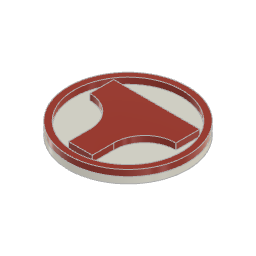
_T.1f97fbe8-ec46-4ea8-aa97-27b6090c93b7 (Autodesk Fusion 360 design; units mm, degrees)
Autodesk Fusion 360 part; units mm, degrees
sketch "Sketch1" plane through (0, 0, 0) normal (0, 0, 1) x (1, 0, 0)
  circle A0 centre (0, 0) radius 15.875
  circle A1 centre (0, 0) radius 14.2875
  line L0 (3.175, -12.7) -> (0, -12.7)
  line L1 (0, -12.7) -> (-3.175, -12.7)
  line L2 (-3.175, -12.7) -> (3.175, -12.7)
  line L3 (3.175, -12.7) -> (3.175, 3.6501)
  line L4 (3.175, 3.6501) -> (-3.175, 3.6501)
  line L5 (-3.175, 3.6501) -> (-3.175, -12.7)
  line L6 (-11.43, 7.62) -> (11.4939, 7.62)
  line L7 (11.4939, 7.62) -> (11.4939, 1.27)
  line L8 (11.4939, 1.27) -> (-11.43, 1.27)
  line L9 (-11.43, 1.27) -> (-11.43, 7.62)
  line L10 (-11.43, 1.27) -> (0.2443, 1.27) construction
  arc A2 (-3.175, -6.985) -> (-11.43, 1.27) centre (-11.43, -6.985) ccw
  line L11 (0, -12.7) -> (0, -11.684)
  arc A3 (11.43, 1.27) -> (3.175, -6.985) centre (11.43, -6.985) ccw
  dimension "d5" = 3.175
  dimension "d16" = 6.35
  constraint coincident A0.centre A1.centre
  constraint horizontal L0
  constraint horizontal L1
  constraint horizontal L2
  constraint vertical L3
  constraint horizontal L4
  constraint vertical L5
  constraint horizontal L6
  constraint vertical L7
  constraint horizontal L8
  constraint vertical L9
  constraint horizontal L10
  constraint coincident L5 A2.start
  constraint tangent L5 A2
  constraint tangent L8 A2
  constraint perpendicular L1 L11
  constraint symmetric L8.end L11 A3.start
  constraint symmetric A2.start L11 A3.end
  constraint symmetric A2 L11 A3
  measures "d5" distance of L0.end L1.end
  measures "d16" distance of L6 L8
extrude "Extrude1" add sketch "Sketch1" against normal blind 1 contours A0 | A1 | L0 L1 L2 L3 L5 L8 | L3 L8 A3 | L3 L4 L5 L8 | L3 L4 L5 L6 L7 L8 L9 | L5 L8 A2 makes body 1 in component "Base"
extrude "Extrude1'" add sketch "Sketch1" along normal blind 1 separate body makes body 2 at (2.3436, 5.0665, 0) makes body 3 at (15.2335, -1.4985, 0) in component "Top"
scale "Scale1" factors (0.6, 0.6, 1) about (3.175, -6.985, 0) bodies 2 3 in component "Top"
scale "Scale1'" factors (0.6, 0.6, 1) about (3.175, -6.985, 0) bodies 1 in component "Base"
component "Base" placed x (1, 0, 0) y (0, 1, 0) z (0, 0, 1) at (0, 0, 0)
component "Top" placed x (1, 0, 0) y (0, 1, 0) z (0, 0, 1) at (0, 0, 0)
